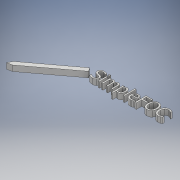
# Autodesk Inventor part: foc
Saved by Autodesk Inventor 2017 (Build 210142000, 142)
## iProperties
Created: 2021-02-26
Part Number: foc
Material: Generic
Document SubType Name: Modeling
Designer: paulg
Density: 1 g/cm^3
Appearance: Default
Author: paulg
Autodesk Inventor part; units mm, degrees
ref_plane "YZ Plane" through (0, 0, 0) normal (1, 0, 0) x (0, 1, 0)
ref_plane "XZ Plane" through (0, 0, 0) normal (0, 1, 0) x (-1, 0, 0)
ref_plane "XY Plane" through (0, 0, 0) normal (0, 0, 1) x (1, 0, 0)
sketch "Sketch1" plane through (0, 0, 0) normal (0, 0, 1) x (1, 0, 0)
  line L0 (-0.0217, 0.1086) -> (142.61, 0.1086) construction
  line L1 (142.61, 0.1086) -> (142.61, -1.7562) construction
  line L2 (142.61, -1.7562) -> (-0.0217, -1.7562) construction
  line L3 (-0.0217, -1.7562) -> (-0.0217, 0.1086) construction
  line L4 (-41.7116, -36.1087) -> (-2.9577, -7.16)
  line L5 (-2.9577, -7.16) -> (-5.3043, -4.0186)
  line L6 (-5.3043, -4.0186) -> (-44.0582, -32.9673)
  line L7 (-44.0582, -32.9673) -> (-41.7116, -36.1087)
  line L8 (-41.7116, -36.1087) -> (-5.3043, -4.0186) construction
  line L9 (-2.9577, -7.16) -> (-44.0582, -32.9673) construction
  line L10 (-44.0582, -32.9673) -> (-46.1916, -37.008)
  line L11 (-46.1916, -37.008) -> (-41.7116, -36.1087)
  line L12 (-46.1916, -37.008) -> (-42.8849, -34.538) construction
  spline S0 degree 2 poles (3.7789, -10.5153) (2.693, -10.5153) (1.1695, -10.0615) (0.4969, -9.7374) knots 0 0 0 1 2 2 2
  line L13 (0.4969, -9.7374) -> (0.4969, -8.068)
  line L14 (0.4969, -8.068) -> (0.5942, -8.068)
  spline S1 degree 2 poles (0.5942, -8.068) (1.2506, -8.6839) (2.9118, -9.3646) (3.6817, -9.3646) knots 0 0 0 1 2 2 2
  spline S2 degree 2 poles (3.6817, -9.3646) (4.7838, -9.3646) (5.9102, -8.4489) (5.9102, -7.6952) knots 0 0 0 1 2 2 2
  spline S3 degree 2 poles (5.9102, -7.6952) (5.9102, -7.0956) (5.3186, -6.35) (4.6784, -6.1636) knots 0 0 0 1 2 2 2
  spline S4 degree 2 poles (4.6784, -6.1636) (4.2165, -6.034) (3.4467, -5.8557) (2.8713, -5.7098) knots 0 0 0 1 2 2 2
  spline S5 degree 2 poles (2.8713, -5.7098) (2.3527, -5.5721) (1.5342, -5.1588) (1.2181, -4.8265) knots 0 0 0 1 2 2 2
  spline S6 degree 2 poles (1.2181, -4.8265) (0.9102, -4.4943) (0.5698, -3.6029) (0.5698, -3.0194) knots 0 0 0 1 2 2 2
  spline S7 degree 2 poles (0.5698, -3.0194) (0.5698, -1.8038) (2.4661, -0.1588) (3.9329, -0.1588) knots 0 0 0 1 2 2 2
  spline S8 degree 2 poles (3.9329, -0.1588) (4.7757, -0.1588) (6.2668, -0.491) (6.907, -0.8071) knots 0 0 0 1 2 2 2
  line L15 (6.907, -0.8071) -> (6.907, -2.3954)
  line L16 (6.907, -2.3954) -> (6.8097, -2.3954)
  spline S9 degree 2 poles (6.8097, -2.3954) (6.3316, -1.9578) (4.8405, -1.3095) (4.022, -1.3095) knots 0 0 0 1 2 2 2
  spline S10 degree 2 poles (4.022, -1.3095) (3.0982, -1.3095) (1.9556, -2.1766) (1.9556, -2.8816) knots 0 0 0 1 2 2 2
  spline S11 degree 2 poles (1.9556, -2.8816) (1.9556, -3.5137) (2.6282, -4.2674) (3.2603, -4.4375) knots 0 0 0 1 2 2 2
  spline S12 degree 2 poles (3.2603, -4.4375) (3.6817, -4.551) (4.9053, -4.8427) (5.3105, -4.9643) knots 0 0 0 1 2 2 2
  spline S13 degree 2 poles (5.3105, -4.9643) (6.3397, -5.2803) (7.2959, -6.5526) (7.2959, -7.4845) knots 0 0 0 1 2 2 2
  spline S14 degree 2 poles (7.2959, -7.4845) (7.2959, -8.0761) (6.8178, -9.2106) (6.3883, -9.6077) knots 0 0 0 1 2 2 2
  spline S15 degree 2 poles (6.3883, -9.6077) (5.9102, -10.0453) (4.6946, -10.5153) (3.7789, -10.5153) knots 0 0 0 1 2 2 2
  line L17 (9.8405, -10.3371) -> (8.5763, -10.3371)
  line L18 (8.5763, -10.3371) -> (8.5763, -2.833)
  line L19 (8.5763, -2.833) -> (9.8405, -2.833)
  line L20 (9.8405, -2.833) -> (9.8405, -10.3371)
  line L21 (9.9296, -1.585) -> (8.4953, -1.585)
  line L22 (8.4953, -1.585) -> (8.4953, -0.2722)
  line L23 (8.4953, -0.2722) -> (9.9296, -0.2722)
  line L24 (9.9296, -0.2722) -> (9.9296, -1.585)
  line L25 (20.2052, -10.3371) -> (20.2052, -5.9935)
  spline S16 degree 2 poles (20.2052, -5.9935) (20.2052, -5.4748) (20.1241, -4.5915) (19.9945, -4.3484) knots 0 0 0 1 2 2 2
  spline S17 degree 2 poles (19.9945, -4.3484) (19.8648, -4.081) (19.3705, -3.8217) (18.941, -3.8217) knots 0 0 0 1 2 2 2
  spline S18 degree 2 poles (18.941, -3.8217) (18.552, -3.8217) (17.6606, -4.2998) (17.1906, -4.7536) knots 0 0 0 1 2 2 2
  spline S19 degree 2 poles (17.1906, -4.7536) (17.1987, -4.867) (17.2149, -5.1831) (17.2149, -5.3938) knots 0 0 0 1 2 2 2
  line L26 (17.2149, -5.3938) -> (17.2149, -10.3371)
  line L27 (17.2149, -10.3371) -> (15.9507, -10.3371)
  line L28 (15.9507, -10.3371) -> (15.9507, -5.9935)
  spline S20 degree 2 poles (15.9507, -5.9935) (15.9507, -5.4748) (15.8697, -4.5915) (15.74, -4.3484) knots 0 0 0 1 2 2 2
  spline S21 degree 2 poles (15.74, -4.3484) (15.6104, -4.081) (15.116, -3.8217) (14.6865, -3.8217) knots 0 0 0 1 2 2 2
  spline S22 degree 2 poles (14.6865, -3.8217) (14.2814, -3.8217) (13.3818, -4.3322) (12.9604, -4.7293) knots 0 0 0 1 2 2 2
  line L29 (12.9604, -4.7293) -> (12.9604, -10.3371)
  line L30 (12.9604, -10.3371) -> (11.6963, -10.3371)
  line L31 (11.6963, -10.3371) -> (11.6963, -2.833)
  line L32 (11.6963, -2.833) -> (12.9604, -2.833)
  line L33 (12.9604, -2.833) -> (12.9604, -3.6596)
  spline S23 degree 2 poles (12.9604, -3.6596) (13.4548, -3.1653) (14.4272, -2.6223) (15.0107, -2.6223) knots 0 0 0 1 2 2 2
  spline S24 degree 2 poles (15.0107, -2.6223) (15.6752, -2.6223) (16.7044, -3.2301) (16.9718, -3.9189) knots 0 0 0 1 2 2 2
  spline S25 degree 2 poles (16.9718, -3.9189) (17.5472, -3.2787) (18.6331, -2.6223) (19.2651, -2.6223) knots 0 0 0 1 2 2 2
  spline S26 degree 2 poles (19.2651, -2.6223) (19.7514, -2.6223) (20.5455, -2.9221) (20.8373, -3.2625) knots 0 0 0 1 2 2 2
  spline S27 degree 2 poles (20.8373, -3.2625) (21.1371, -3.6029) (21.4694, -4.6239) (21.4694, -5.3938) knots 0 0 0 1 2 2 2
  line L34 (21.4694, -5.3938) -> (21.4694, -10.3371)
  line L35 (21.4694, -10.3371) -> (20.2052, -10.3371)
  spline S28 degree 2 poles (29.5326, -6.3824) (29.5326, -8.2625) (27.7416, -10.4829) (26.3721, -10.4829) knots 0 0 0 1 2 2 2
  spline S29 degree 2 poles (26.3721, -10.4829) (25.813, -10.4829) (24.954, -10.2236) (24.5083, -9.9562) knots 0 0 0 1 2 2 2
  line L36 (24.5083, -9.9562) -> (24.5083, -13.1004)
  line L37 (24.5083, -13.1004) -> (23.2441, -13.1004)
  line L38 (23.2441, -13.1004) -> (23.2441, -2.833)
  line L39 (23.2441, -2.833) -> (24.5083, -2.833)
  line L40 (24.5083, -2.833) -> (24.5083, -3.6191)
  spline S30 degree 2 poles (24.5083, -3.6191) (24.9783, -3.1896) (26.129, -2.6223) (26.8016, -2.6223) knots 0 0 0 1 2 2 2
  spline S31 degree 2 poles (26.8016, -2.6223) (28.0901, -2.6223) (29.5326, -4.6644) (29.5326, -6.3824) knots 0 0 0 1 2 2 2
  spline S32 degree 2 poles (28.2279, -6.5283) (28.2279, -5.2398) (27.4094, -3.8217) (26.4937, -3.8217) knots 0 0 0 1 2 2 2
  spline S33 degree 2 poles (26.4937, -3.8217) (25.9588, -3.8217) (24.954, -4.2998) (24.5083, -4.6726) knots 0 0 0 1 2 2 2
  line L41 (24.5083, -4.6726) -> (24.5083, -8.9351)
  spline S34 degree 2 poles (24.5083, -8.9351) (25.0026, -9.1701) (25.7076, -9.3484) (26.1614, -9.3484) knots 0 0 0 1 2 2 2
  spline S35 degree 2 poles (26.1614, -9.3484) (27.142, -9.3484) (28.2279, -7.9059) (28.2279, -6.5283) knots 0 0 0 1 2 2 2
  line L42 (32.1339, -10.3371) -> (30.8697, -10.3371)
  line L43 (30.8697, -10.3371) -> (30.8697, 0.1086)
  line L44 (30.8697, 0.1086) -> (32.1339, 0.1086)
  line L45 (32.1339, 0.1086) -> (32.1339, -10.3371)
  spline S36 degree 2 poles (37.2473, -10.5072) (35.4483, -10.5072) (33.471, -8.4894) (33.471, -6.6256) knots 0 0 0 1 2 2 2
  spline S37 degree 2 poles (33.471, -6.6256) (33.471, -4.7941) (35.3916, -2.6223) (36.9394, -2.6223) knots 0 0 0 1 2 2 2
  spline S38 degree 2 poles (36.9394, -2.6223) (37.6363, -2.6223) (38.7141, -3.0275) (39.1112, -3.457) knots 0 0 0 1 2 2 2
  spline S39 degree 2 poles (39.1112, -3.457) (39.5164, -3.8865) (39.9459, -5.1264) (39.9459, -6.0259) knots 0 0 0 1 2 2 2
  line L46 (39.9459, -6.0259) -> (39.9459, -6.7147)
  line L47 (39.9459, -6.7147) -> (34.7514, -6.7147)
  spline S40 degree 2 poles (34.7514, -6.7147) (34.7514, -8.0194) (36.0642, -9.4051) (37.2311, -9.4051) knots 0 0 0 1 2 2 2
  spline S41 degree 2 poles (37.2311, -9.4051) (37.6444, -9.4051) (38.4467, -9.2187) (38.7708, -9.0729) knots 0 0 0 1 2 2 2
  spline S42 degree 2 poles (38.7708, -9.0729) (39.1112, -8.9108) (39.5812, -8.6272) (39.7352, -8.4975) knots 0 0 0 1 2 2 2
  line L48 (39.7352, -8.4975) -> (39.8081, -8.4975)
  line L49 (39.8081, -8.4975) -> (39.8081, -9.8751)
  spline S43 degree 2 poles (39.8081, -9.8751) (39.5893, -9.9643) (38.9248, -10.2236) (38.6655, -10.2965) knots 0 0 0 1 2 2 2
  spline S44 degree 2 poles (38.6655, -10.2965) (38.3008, -10.4019) (37.7011, -10.5072) (37.2473, -10.5072) knots 0 0 0 1 2 2 2
  spline S45 degree 2 poles (38.7141, -5.7503) (38.6979, -5.2398) (38.4872, -4.4943) (38.2846, -4.2431) knots 0 0 0 1 2 2 2
  spline S46 degree 2 poles (38.2846, -4.2431) (38.0658, -3.9594) (37.377, -3.6596) (36.8664, -3.6596) knots 0 0 0 1 2 2 2
  spline S47 degree 2 poles (36.8664, -3.6596) (36.364, -3.6596) (35.659, -3.9594) (35.3672, -4.2512) knots 0 0 0 1 2 2 2
  spline S48 degree 2 poles (35.3672, -4.2512) (35.0836, -4.551) (34.7919, -5.2722) (34.7514, -5.7503) knots 0 0 0 1 2 2 2
  line L50 (34.7514, -5.7503) -> (38.7141, -5.7503)
  line L51 (47.304, -1.5202) -> (42.6525, -1.5202)
  line L52 (42.6525, -1.5202) -> (42.6525, -4.3403)
  line L53 (42.6525, -4.3403) -> (47.1096, -4.3403)
  line L54 (47.1096, -4.3403) -> (47.1096, -5.5234)
  line L55 (47.1096, -5.5234) -> (42.6525, -5.5234)
  line L56 (42.6525, -5.5234) -> (42.6525, -10.3371)
  line L57 (42.6525, -10.3371) -> (41.3235, -10.3371)
  line L58 (41.3235, -10.3371) -> (41.3235, -0.3371)
  line L59 (41.3235, -0.3371) -> (47.304, -0.3371)
  line L60 (47.304, -0.3371) -> (47.304, -1.5202)
  spline S49 degree 2 poles (55.5698, -1.4797) (56.1371, -2.1442) (56.7692, -4.0891) (56.7692, -5.3371) knots 0 0 0 1 2 2 2
  spline S50 degree 2 poles (56.7692, -5.3371) (56.7692, -6.5526) (56.1533, -8.5218) (55.5698, -9.1863) knots 0 0 0 1 2 2 2
  spline S51 degree 2 poles (55.5698, -9.1863) (54.954, -9.8833) (53.3251, -10.5478) (52.3446, -10.5478) knots 0 0 0 1 2 2 2
  spline S52 degree 2 poles (52.3446, -10.5478) (51.3316, -10.5478) (49.7108, -9.8589) (49.1193, -9.1863) knots 0 0 0 1 2 2 2
  spline S53 degree 2 poles (49.1193, -9.1863) (48.5439, -8.5218) (47.928, -6.5688) (47.928, -5.3371) knots 0 0 0 1 2 2 2
  spline S54 degree 2 poles (47.928, -5.3371) (47.928, -4.081) (48.552, -2.1685) (49.1274, -1.4797) knots 0 0 0 1 2 2 2
  spline S55 degree 2 poles (49.1274, -1.4797) (49.7108, -0.8152) (51.3397, -0.1264) (52.3446, -0.1264) knots 0 0 0 1 2 2 2
  spline S56 degree 2 poles (52.3446, -0.1264) (53.3656, -0.1264) (55.0026, -0.8395) (55.5698, -1.4797) knots 0 0 0 1 2 2 2
  spline S57 degree 2 poles (55.3835, -5.3371) (55.3835, -4.3484) (54.954, -2.8168) (54.565, -2.3144) knots 0 0 0 1 2 2 2
  spline S58 degree 2 poles (54.565, -2.3144) (54.1679, -1.7957) (53.0496, -1.2771) (52.3527, -1.2771) knots 0 0 0 1 2 2 2
  spline S59 degree 2 poles (52.3527, -1.2771) (51.6314, -1.2771) (50.5455, -1.7795) (50.1322, -2.3144) knots 0 0 0 1 2 2 2
  spline S60 degree 2 poles (50.1322, -2.3144) (49.7352, -2.8249) (49.3138, -4.3646) (49.3138, -5.3371) knots 0 0 0 1 2 2 2
  spline S61 degree 2 poles (49.3138, -5.3371) (49.3138, -7.3063) (50.9669, -9.397) (52.3527, -9.397) knots 0 0 0 1 2 2 2
  spline S62 degree 2 poles (52.3527, -9.397) (53.7384, -9.397) (55.3835, -7.3063) (55.3835, -5.3371) knots 0 0 0 1 2 2 2
  spline S63 degree 2 poles (62.1339, -10.5153) (61.1614, -10.5153) (59.5164, -9.8589) (58.9167, -9.2025) knots 0 0 0 1 2 2 2
  spline S64 degree 2 poles (58.9167, -9.2025) (58.317, -8.5542) (57.6606, -6.6093) (57.6606, -5.3452) knots 0 0 0 1 2 2 2
  spline S65 degree 2 poles (57.6606, -5.3452) (57.6606, -4.0891) (58.3008, -2.2252) (58.9086, -1.5364) knots 0 0 0 1 2 2 2
  spline S66 degree 2 poles (58.9086, -1.5364) (59.5083, -0.8638) (61.1452, -0.1588) (62.1582, -0.1588) knots 0 0 0 1 2 2 2
  spline S67 degree 2 poles (62.1582, -0.1588) (62.6606, -0.1588) (63.5439, -0.3046) (63.9167, -0.4181) knots 0 0 0 1 2 2 2
  spline S68 degree 2 poles (63.9167, -0.4181) (64.2408, -0.5234) (64.9134, -0.8233) (65.2457, -1.0016) knots 0 0 0 1 2 2 2
  line L61 (65.2457, -1.0016) -> (65.2457, -2.6061)
  line L62 (65.2457, -2.6061) -> (65.1403, -2.6061)
  spline S69 degree 2 poles (65.1403, -2.6061) (64.9621, -2.444) (64.411, -1.9902) (64.0139, -1.7714) knots 0 0 0 1 2 2 2
  spline S70 degree 2 poles (64.0139, -1.7714) (63.6331, -1.5607) (62.7335, -1.2933) (62.1501, -1.2933) knots 0 0 0 1 2 2 2
  spline S71 degree 2 poles (62.1501, -1.2933) (61.5099, -1.2933) (60.3672, -1.82) (59.9378, -2.3225) knots 0 0 0 1 2 2 2
  spline S72 degree 2 poles (59.9378, -2.3225) (59.5164, -2.833) (59.0463, -4.3808) (59.0463, -5.3452) knots 0 0 0 1 2 2 2
  spline S73 degree 2 poles (59.0463, -5.3452) (59.0463, -6.3743) (59.5407, -7.8573) (59.9702, -8.3679) knots 0 0 0 1 2 2 2
  spline S74 degree 2 poles (59.9702, -8.3679) (60.3916, -8.8622) (61.518, -9.3646) (62.1501, -9.3646) knots 0 0 0 1 2 2 2
  spline S75 degree 2 poles (62.1501, -9.3646) (62.7254, -9.3646) (63.706, -9.081) (64.0869, -8.8703) knots 0 0 0 1 2 2 2
  spline S76 degree 2 poles (64.0869, -8.8703) (64.4515, -8.6596) (64.9945, -8.222) (65.1484, -8.068) knots 0 0 0 1 2 2 2
  line L63 (65.1484, -8.068) -> (65.2457, -8.068)
  line L64 (65.2457, -8.068) -> (65.2457, -9.6563)
  spline S77 degree 2 poles (65.2457, -9.6563) (64.9134, -9.8103) (64.33, -10.0939) (63.9167, -10.2236) knots 0 0 0 1 2 2 2
  spline S78 degree 2 poles (63.9167, -10.2236) (63.4791, -10.3695) (62.7335, -10.5153) (62.1339, -10.5153) knots 0 0 0 1 2 2 2
  point P0 (0, 0)
  point P1 (-23.5079, -20.0636)
  constraints: 18 end point, 3 midpoint, 3 parallel, 1 perpendicular, 2 other
extrude "Extrusion1" add sketch "Sketch1" along normal blind 5
body "Solid1"
